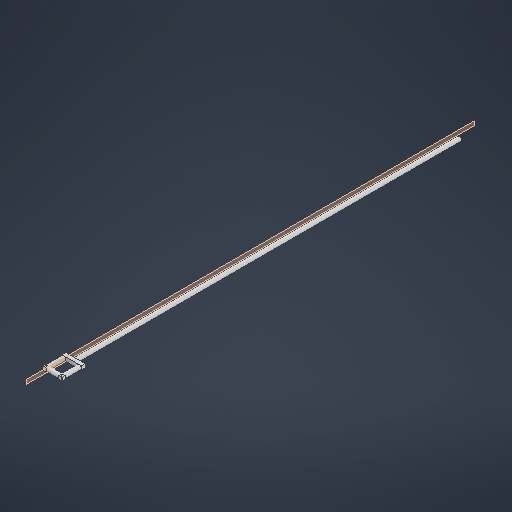
# Autodesk Inventor part: táhlo
Saved by Autodesk Inventor 2026 (Build 300175050, 175E)
## iProperties
Created: 2026-03-20
Part Number: táhlo
Material: Všeobecné
Document SubType Name: Modeling
Designer: marti
Density: 1 g/cm^3
Appearance: Výchozí
Author: marti
Autodesk Inventor part; units mm, degrees
ref_plane "YZ Plane" through (0, 0, 0) normal (1, 0, 0) x (0, 1, 0)
ref_plane "XZ Plane" through (0, 0, 0) normal (0, 1, 0) x (-1, 0, 0)
ref_plane "XY Plane" through (0, 0, 0) normal (0, 0, 1) x (1, 0, 0)
sketch "Náčrt1" plane through (0, 0, 0) normal (0, 0, 1) x (1, 0, 0)
  circle A0 centre (0, 0) radius 1
  dimension "d0" = 2
  constraints: 1 centre point, 1 coincident
  measures "d0" diameter of A0
extrude "Vysunutí1" add sketch "Náčrt1" along normal blind 200
sketch "Náčrt2" plane through (0, 0, 200) normal (0, 0, 1) x (1, 0, 0)
  line L0 (-5, 1) -> (5, 1)
  line L1 (5, 1) -> (5, -1)
  line L2 (5, -1) -> (-5, -1)
  line L3 (-5, -1) -> (-5, 1)
  line L4 (-7, 0) -> (7, 0) projected
  line L5 (0, 1.4) -> (0, -1.4) projected
  point P0 (0, 0)
  dimension "d3" = 10
  constraints: 8 end point, 2 parallel, 1 horizontal, 1 perpendicular, 2 other
  measures "d3" distance of L1.end L2.end
extrude "Vysunutí2" add sketch "Náčrt2" along normal blind 2
sketch "Náčrt3" plane through (0, 0, 202) normal (0, 0, 1) x (1, 0, 0)
  line L0 (-5, -1) -> (5, -1) projected
  line L1 (5, -1) -> (5, 1) projected
  line L2 (5, 1) -> (-5, 1) projected
  line L3 (-5, 1) -> (-5, -1) projected
  circle A0 centre (-4, 0) radius 1
  circle A1 centre (4, 0) radius 1
  point P0 (0, 0)
  constraints: 6 tangent, 2 centre point
extrude "Vysunutí3" add sketch "Náčrt3" along normal blind 10 contours A0 | A1
ref_plane "Pracovní rovina1" through (-3, 0, 202) normal (1, 0, 0) x (0, 0, -1)
sketch "Náčrt4" plane through (-3, 0, 202) normal (1, 0, 0) x (0, 0, -1)
  line L0 (-10, 1) -> (-10, -1) projected
  line L1 (0, 1) -> (0, -1) projected
  line L2 (0, 0) -> (0, 1) projected
  line L3 (0, -1) -> (0, 0) projected
  line L4 (0, 1) -> (-10, 1) projected
  line L5 (0, -1) -> (-10, -1) projected
  circle A0 centre (-9, 0) radius 1
  point P0 (202, 0)
  constraints: 3 tangent, 1 centre point
extrude "Vysunutí4" add sketch "Náčrt4" along normal blind 8 and the other way blind 2 contours A0
